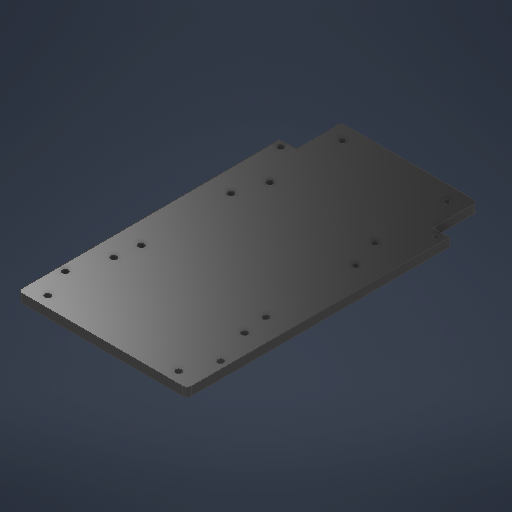
# Autodesk Inventor part: BASE_ELETRONICA
Saved by Autodesk Inventor 2027.1 (Build 311270010, 270A)
## iProperties
Created: 2026-08-16
Part Number: BASE_ELETRONICA
Material: Genérico
Document SubType Name: Modeling
Designer: Evellyn
Density: 1 g/cm^3
Appearance: Padrão
Author: Evellyn
Autodesk Inventor part; units mm, degrees
ref_plane "YZ Plane" through (0, 0, 0) normal (1, 0, 0) x (0, 1, 0)
ref_plane "XZ Plane" through (0, 0, 0) normal (0, 1, 0) x (-1, 0, 0)
ref_plane "XY Plane" through (0, 0, 0) normal (0, 0, 1) x (1, 0, 0)
sketch "Esboço1" plane through (0, 0, 0) normal (0, 1, 0) x (-1, 0, 0)
  line L0 (-30.2, -70) -> (30.2, -70)
  line L1 (40, -48.6559) -> (40, 73)
  line L2 (38, 75) -> (-38, 75)
  line L3 (-40, 73) -> (-40, -48.6559)
  line L4 (-40, -70) -> (40, 75) construction
  line L5 (40, -70) -> (-40, 75) construction
  line L6 (0, 77.1224) -> (0, -77.4589)
  line L7 (55.8999, -0.1682) -> (-68.6929, -0.1682)
  arc A0 (40, 73) -> (38, 75) centre (38, 73) ccw
  arc A1 (-38, 75) -> (-40, 73) centre (-38, 73) ccw
  line L8 (-33, 36.5618) -> (33, 36.5618)
  line L9 (33, 36.5618) -> (33, 71.9618)
  line L10 (33, 71.9618) -> (-33, 71.9618)
  line L11 (-33, 71.9618) -> (-33, 36.5618)
  line L12 (-33, 36.5618) -> (33, 71.9618) construction
  line L13 (33, 36.5618) -> (-33, 71.9618) construction
  line L14 (-35.75, -19.4382) -> (35.75, -19.4382)
  line L15 (35.75, -19.4382) -> (35.75, 31.5618)
  line L16 (35.75, 31.5618) -> (-35.75, 31.5618)
  line L17 (-35.75, 31.5618) -> (-35.75, -19.4382)
  line L18 (-35.75, -19.4382) -> (35.75, 31.5618) construction
  line L19 (35.75, -19.4382) -> (-35.75, 31.5618) construction
  line L20 (-27.1, -67.2382) -> (27.1, -67.2382)
  line L21 (29.1, -65.2382) -> (29.1, -26.4382)
  line L22 (27.1, -24.4382) -> (-27.1, -24.4382)
  line L23 (-29.1, -26.4382) -> (-29.1, -65.2382)
  line L24 (-29.1, -67.2382) -> (29.1, -24.4382) construction
  line L25 (29.1, -67.2382) -> (-29.1, -24.4382) construction
  arc A2 (29.1, -26.4382) -> (27.1, -24.4382) centre (27.1, -26.4382) ccw
  arc A3 (27.1, -67.2382) -> (29.1, -65.2382) centre (27.1, -65.2382) ccw
  arc A4 (-29.1, -65.2382) -> (-27.1, -67.2382) centre (-27.1, -65.2382) ccw
  arc A5 (-27.1, -24.4382) -> (-29.1, -26.4382) centre (-27.1, -26.4382) ccw
  circle A6 centre (30.85, 69.8118) radius 1.35
  circle A7 centre (-30.85, 69.8118) radius 1.35
  circle A8 centre (30.85, 38.7118) radius 1.35
  circle A9 centre (-30.85, 38.7118) radius 1.35
  circle A10 centre (29.4, 27.2118) radius 1.35
  circle A11 centre (-29.4, 27.2118) radius 1.35
  circle A12 centre (29.4, -15.0882) radius 1.35
  circle A13 centre (-29.4, -15.0882) radius 1.35
  line L26 (29.1, -45.8382) -> (-29.1, -45.8382)
  circle A14 centre (24.75, -28.7882) radius 1.35
  circle A15 centre (-24.75, -28.7882) radius 1.35
  circle A16 centre (24.75, -62.8882) radius 1.35
  circle A17 centre (-24.75, -62.8882) radius 1.35
  circle A18 centre (36.65, 55.7814) radius 1.35
  circle A19 centre (-36.65, 55.7814) radius 1.35
  circle A20 centre (36.65, -45.8382) radius 1.35
  circle A21 centre (-36.65, -45.8382) radius 1.35
  line L27 (32.2, -52.4162) -> (32.2, -68)
  line L28 (-32.2, -52.4162) -> (-32.2, -68)
  arc A22 (-32.2, -68) -> (-30.2, -70) centre (-30.2, -68) ccw
  arc A23 (30.2, -70) -> (32.2, -68) centre (30.2, -68) ccw
  line L29 (40, -48.6559) -> (32.2, -48.6559)
  line L30 (32.2, -48.6559) -> (32.2, -52.4162)
  line L31 (-40, -48.6559) -> (-32.2, -48.6559)
  line L32 (-32.2, -48.6559) -> (-32.2, -52.4162)
  point P0 (39.576, -69.2314)
  point P1 (0, 54.2618)
  point P2 (0, 6.0618)
  point P3 (0, -45.8382)
  point P4 (32.2, -70)
  point P5 (-32.2, -70)
  dimension "d8" = 2
  dimension "d13" = 35.4
  dimension "d14" = 71.5
  dimension "d16" = 58.2
  dimension "d18" = 5
  dimension "d19" = 5
  dimension "d21" = 2.7
  dimension "d22" = 0.8
  dimension "d23" = 0.8
  dimension "d24" = 2.7
  dimension "d25" = 3
  dimension "d26" = 5
  dimension "d27" = 2.7
  dimension "d28" = 3
  dimension "d30" = 3
  dimension "d33" = 2.7
  dimension "d34" = 2
  dimension "d36" = 2
  dimension "d45" = 3.35
  dimension "d46" = 17.2186
  dimension "d47" = 2
  dimension "d48" = 2
  constraints: 66 end point, 24 centre point, 24 point on line, 16 point on circle, 16 tangent, 9 symmetric about line, 8 midpoint, 8 parallel, 7 horizontal, 7 perpendicular, 4 equal radius, 1 vertical, 7 other
  measures "d8" radius of A0
  measures "d13" distance of L9.end L8.end
  measures "d14" distance of L16.end L15.end
  measures "d16" distance of L25.end L24.end
  measures "d18" distance between parallel lines of L16 L8
  measures "d19" distance between parallel lines of L14 L22
  measures "d21" diameter of A6
  measures "d22" distance edge to line of A6 L9
  measures "d23" distance edge to line of A6 L10
  measures "d24" diameter of A10
  measures "d25" distance edge to line of A10 L16
  measures "d26" distance edge to line of A10 L15
  measures "d27" diameter of A14
  measures "d28" distance edge to line of A14 L21
  measures "d30" distance edge to line of A14 L22
  measures "d33" diameter of A18
  measures "d34" distance edge to line of A18 L1
  measures "d36" distance edge to line of A20 L1
  measures "d45" distance from line of A21.centre L3
  measures "d46" vertical distance of A1.centre A19.centre
  measures "d47" radius of A22
  measures "d48" radius of A23
extrude "Extrusão1" add sketch "Esboço1" along normal blind 4 contours A22 L28 L32 L31 L3 L7 L17 L14 L6 L22 A5 L23 A4 L20 L0 | L6 L20 A3 L21 A2 L22 L14 L15 L7 L1 L29 L30 L27 A23 L0 | L20 A4 L23 L26 L6 | L6 L26 L21 A3 L20 | L26 L23 A5 L22 L6 | L6 L22 A2 L21 L26 | L14 L17 L7 L6 | L6 L7 L15 L14 | L3 A1 L2 L6 L10 L11 L8 L16 L17 L7 | L7 L17 L16 L6 | L6 L16 L15 L7 | L7 L15 L16 L6 L8 L9 L10 L2 A0 L1 | L8 L11 L10 L6 | L6 L10 L9 L8 | A18 | A19 | A20 | A21
hole "Furo1" at (36.65, 0, -45.8382) at (-36.65, 0, -45.8382) at (-36.65, 0, 55.7814) at (36.65, 0, 55.7814) direction (0, 1, 0) diameter 2.7 end through all
